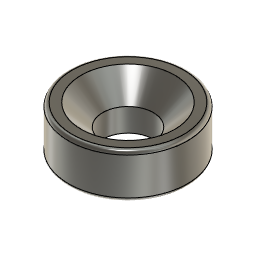
FlintZone RC 1.0 (Autodesk Fusion 360 archive; units mm, degrees)
design "Magnet 8x3"
Autodesk Fusion 360 part; units mm, degrees
sketch "Sketch1" plane through (0, 0, 0) normal (0, 0, 1) x (1, 0, 0)
  circle A0 centre (0, 0) radius 4
  dimension "d1" = 8
  constraint coincident A0.centre origin
  measures "d1" diameter of A0
extrude "Extrude1" add sketch "Sketch1" along normal blind 3
hole "Hole1" at (0, 0, 3) direction (0, 0, -1) diameter 3.4 depth 8 tip angle 118 countersink diameter 6.3 countersink angle 90
fillet "Fillet1" radius 0.25 2 edges at (-3.7293, -1.4465, 0) (-3.7293, -1.4465, 3)
